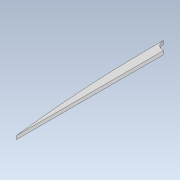
# Autodesk Inventor part: aileron_static
Saved by Autodesk Inventor 2020 (Build 240168000, 168)
## iProperties
Created: 2020-09-10
Part Number: aileron_static
Material: Generic
Document SubType Name: Modeling
Designer: Admin
Density: 1 g/cm^3
Appearance: Default
Author: Admin
Autodesk Inventor part; units mm, degrees
ref_plane "YZ Plane" through (0, 0, 0) normal (1, 0, 0) x (0, 1, 0)
ref_plane "XZ Plane" through (0, 0, 0) normal (0, 1, 0) x (-1, 0, 0)
ref_plane "XY Plane" through (0, 0, 0) normal (0, 0, 1) x (1, 0, 0)
sketch "Sketch1" plane through (0, 0, 0) normal (0, 1, 0) x (-1, 0, 0)
  line L0 (0, 0) -> (0, -83)
  arc A0 (5, -88) -> (0, -83) centre (0, -88) ccw
  line L1 (5, -83) -> (5, -88)
  arc A1 (5, -83) -> (0, 0) centre (-686.4, -83) ccw
  dimension "d3" = 0
  dimension "d4" = 0
  dimension "d5" = 5
  constraints: 4 end point, 4 point on circle, 2 centre point, 1 coincident
  measures "d3" distance from line of A0.centre L0
  measures "d4" vertical distance of A0.centre L1.end
  measures "d5" radius of A0
extrude "Extrusion1" add sketch "Sketch1" along normal blind 2
body "Solid1"
